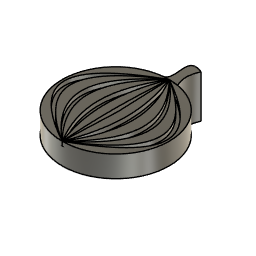
pumpkin (Autodesk Fusion 360 design; units mm, degrees)
Autodesk Fusion 360 part; units mm, degrees
sketch "Sketch1" plane through (0, 0, 0) normal (0, 0, 1) x (1, 0, 0)
  circle A0 centre (0, 0) radius 25
  constraint coincident A0.centre origin
extrude "Extrude1" add sketch "Sketch1" along normal blind 10 makes body 1
sketch "Sketch2" plane through (0, 0, 10) normal (0, 0, 1) x (-1, 0, 0)
  circle A0 centre (0, 0) radius 25
  spline S0 degree 5 poles (0, -25) (-0.3792, -24) (-1.1046, -22) (-2.0933, -19) (-3.2095, -15) (-4.2453, -10) (-4.8894, -5) (-5.11, 0) (-4.8894, 5) (-4.2453, 10) (-3.2095, 15) (-2.0933, 19) (-1.1046, 22) (-0.3792, 24) (0, 25) knots 0 0 0 0 0 0 0.1 0.2 0.3 0.4 0.5 0.6 0.7 0.8 0.9 1 1 1 1 1 1
  spline S1 degree 5 poles (0, -25) (0.3792, -24) (1.1046, -22) (2.0933, -19) (3.2095, -15) (4.2453, -10) (4.8894, -5) (5.11, 0) (4.8894, 5) (4.2453, 10) (3.2095, 15) (2.0933, 19) (1.1046, 22) (0.3792, 24) (0, 25) knots 0 0 0 0 0 0 0.1 0.2 0.3 0.4 0.5 0.6 0.7 0.8 0.9 1 1 1 1 1 1
  spline S2 degree 5 poles (0, -25) (-0.6068, -24) (-1.7674, -22) (-3.3492, -19) (-5.1352, -15) (-6.7925, -10) (-7.8231, -5) (-8.176, 0) (-7.8231, 5) (-6.7925, 10) (-5.1352, 15) (-3.3492, 19) (-1.7674, 22) (-0.6068, 24) (0, 25) knots 0 0 0 0 0 0 0.1 0.2 0.3 0.4 0.5 0.6 0.7 0.8 0.9 1 1 1 1 1 1
  spline S3 degree 5 poles (0, -25) (0.6068, -24) (1.7674, -22) (3.3492, -19) (5.1352, -15) (6.7925, -10) (7.8231, -5) (8.176, 0) (7.8231, 5) (6.7925, 10) (5.1352, 15) (3.3492, 19) (1.7674, 22) (0.6068, 24) (0, 25) knots 0 0 0 0 0 0 0.1 0.2 0.3 0.4 0.5 0.6 0.7 0.8 0.9 1 1 1 1 1 1
  spline S4 degree 5 poles (0, -25) (-0.986, -24) (-2.8719, -22) (-5.4425, -19) (-8.3448, -15) (-11.0378, -10) (-12.7126, -5) (-13.2859, 0) (-12.7126, 5) (-11.0378, 10) (-8.3448, 15) (-5.4425, 19) (-2.8719, 22) (-0.986, 24) (0, 25) knots 0 0 0 0 0 0 0.1 0.2 0.3 0.4 0.5 0.6 0.7 0.8 0.9 1 1 1 1 1 1
  spline S5 degree 5 poles (0, -25) (-1.2136, -24) (-3.5347, -22) (-6.6985, -19) (-10.2705, -15) (-13.585, -10) (-15.6462, -5) (-16.3519, 0) (-15.6462, 5) (-13.585, 10) (-10.2705, 15) (-6.6985, 19) (-3.5347, 22) (-1.2136, 24) (0, 25) knots 0 0 0 0 0 0 0.1 0.2 0.3 0.4 0.5 0.6 0.7 0.8 0.9 1 1 1 1 1 1
  spline S6 degree 5 poles (0, -25) (-1.5928, -24) (-4.6393, -22) (-8.7918, -19) (-13.48, -15) (-17.8303, -10) (-20.5357, -5) (-21.4619, 0) (-20.5357, 5) (-17.8303, 10) (-13.48, 15) (-8.7918, 19) (-4.6393, 22) (-1.5928, 24) (0, 25) knots 0 0 0 0 0 0 0.1 0.2 0.3 0.4 0.5 0.6 0.7 0.8 0.9 1 1 1 1 1 1
  spline S7 degree 5 poles (0, -25) (-1.8203, -24) (-5.3021, -22) (-10.0477, -19) (-15.4057, -15) (-20.3775, -10) (-23.4693, -5) (-24.5279, 0) (-23.4693, 5) (-20.3775, 10) (-15.4057, 15) (-10.0477, 19) (-5.3021, 22) (-1.8203, 24) (0, 25) knots 0 0 0 0 0 0 0.1 0.2 0.3 0.4 0.5 0.6 0.7 0.8 0.9 1 1 1 1 1 1
  spline S8 degree 5 poles (0, -25) (0.986, -24) (2.8719, -22) (5.4425, -19) (8.3448, -15) (11.0378, -10) (12.7126, -5) (13.2859, 0) (12.7126, 5) (11.0378, 10) (8.3448, 15) (5.4425, 19) (2.8719, 22) (0.986, 24) (0, 25) knots 0 0 0 0 0 0 0.1 0.2 0.3 0.4 0.5 0.6 0.7 0.8 0.9 1 1 1 1 1 1
  spline S9 degree 5 poles (0, -25) (1.2136, -24) (3.5347, -22) (6.6985, -19) (10.2705, -15) (13.585, -10) (15.6462, -5) (16.3519, 0) (15.6462, 5) (13.585, 10) (10.2705, 15) (6.6985, 19) (3.5347, 22) (1.2136, 24) (0, 25) knots 0 0 0 0 0 0 0.1 0.2 0.3 0.4 0.5 0.6 0.7 0.8 0.9 1 1 1 1 1 1
  spline S10 degree 5 poles (0, -25) (1.5928, -24) (4.6393, -22) (8.7918, -19) (13.48, -15) (17.8303, -10) (20.5357, -5) (21.4619, 0) (20.5357, 5) (17.8303, 10) (13.48, 15) (8.7918, 19) (4.6393, 22) (1.5928, 24) (0, 25) knots 0 0 0 0 0 0 0.1 0.2 0.3 0.4 0.5 0.6 0.7 0.8 0.9 1 1 1 1 1 1
  spline S11 degree 5 poles (0, -25) (1.8203, -24) (5.3021, -22) (10.0477, -19) (15.4057, -15) (20.3775, -10) (23.4693, -5) (24.5279, 0) (23.4693, 5) (20.3775, 10) (15.4057, 15) (10.0477, 19) (5.3021, 22) (1.8203, 24) (0, 25) knots 0 0 0 0 0 0 0.1 0.2 0.3 0.4 0.5 0.6 0.7 0.8 0.9 1 1 1 1 1 1
  line L0 (0, 25) -> (-1, 0)
  line L1 (-1, 0) -> (0, -25)
  spline S12 degree 5 poles (0, -25) (0.0758, -24) (0.2209, -22) (0.4187, -19) (0.6419, -15) (0.8491, -10) (0.9779, -5) (1.022, 0) (0.9779, 5) (0.8491, 10) (0.6419, 15) (0.4187, 19) (0.2209, 22) (0.0758, 24) (0, 25) knots 0 0 0 0 0 0 0.1 0.2 0.3 0.4 0.5 0.6 0.7 0.8 0.9 1 1 1 1 1 1
  point P0 (-5, 0)
  point P1 (5, 0)
  point P2 (-8, 0)
  point P3 (8, 0)
  point P4 (-13, 0)
  point P5 (-16, 0)
  point P6 (-21, 0)
  point P7 (-24, 0)
  point P8 (13, 0)
  point P9 (16, 0)
  point P10 (21, 0)
  point P11 (24, 0)
  point P12 (1, 0)
  constraint coincident A0 S0.start
  constraint coincident A0 S0.end
extrude "Extrude2" cut sketch "Sketch2" against normal blind 2 contours S1 S3 | S0 S2 | S4 S5 | S6 S7 | S8 S9 | S10 S11 | L0 L1 S12 bodies 1
sketch "Sketch3" plane through (0, 0, 10) normal (0, 0, 1) x (-1, 0, 0)
  spline S0 degree 5 poles (0, 25) (1.8203, 24) (5.3021, 22) (10.0477, 19) (15.4057, 15) (20.3775, 10) (23.4693, 5) (24.5279, 0) (23.4693, -5) (20.3775, -10) (15.4057, -15) (10.0477, -19) (5.3021, -22) (1.8203, -24) (0, -25) knots -1 -1 -1 -1 -1 -1 -0.9 -0.8 -0.7 -0.6 -0.5 -0.4 -0.3 -0.2 -0.1 0 0 0 0 0 0
  arc A0 (0, -25) -> (0, 25) centre (0, 0) ccw
  line L0 (0, 0) -> (25, 0) construction
  line L1 (0, 0) -> (-25, 0) construction
  spline S1 degree 5 poles (4.3412, -24.6202) (4.0652, -24.5975) (3.5414, -24.583) (2.8403, -24.6537) (2.076, -24.9343) (1.4065, -25.597) (1.0139, -26.5616) (0.8704, -27.797) (0.9159, -29.2361) (1.0635, -30.7818) (1.2128, -32.3223) (1.2603, -33.7424) (1.1111, -34.9361) (0.6892, -35.8191) (-0.048, -36.3442) (-1.1179, -36.4921) (-2.2421, -36.3066) (-3.2341, -35.9988) (-3.9612, -35.7192) (-4.3412, -35.5608) knots 0 0 0 0 0 0 0.066667 0.133333 0.2 0.266667 0.333333 0.4 0.466667 0.533333 0.6 0.666667 0.733333 0.8 0.866667 0.933333 1 1 1 1 1 1
  spline S2 degree 5 poles (-4.3412, -35.5608) (-4.2397, -35.3378) (-4.0455, -34.8923) (-3.7808, -34.225) (-3.4816, -33.3376) (-3.2037, -32.2321) (-3.0304, -31.131) (-2.9705, -30.0345) (-3.0288, -28.9428) (-3.2011, -27.8558) (-3.4789, -26.7731) (-3.7786, -25.9101) (-4.0443, -25.2645) (-4.2393, -24.8348) (-4.3412, -24.6202) knots 0 0 0 0 0 0 0.1 0.2 0.3 0.4 0.5 0.6 0.7 0.8 0.9 1 1 1 1 1 1
  line L2 (4.3412, -24.6202) -> (0, -25)
  line L3 (0, -25) -> (-4.3412, -24.6202)
  point P0 (1, -27)
  point P1 (1, -35)
  point P2 (-3, -30)
  constraint horizontal L0
  constraint coincident A0.centre L0.start
  constraint horizontal L1
  constraint coincident S0.end A0.start
extrude "Extrude3" add sketch "Sketch3" against normal blind 20 separate body contours A0 S1 S2 L3 makes body 2
